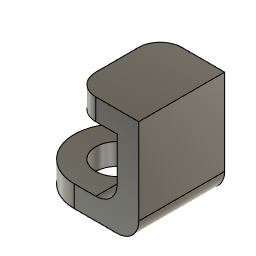
Practice3 (Autodesk Fusion 360 design; units mm, degrees)
Autodesk Fusion 360 part; units mm, degrees
sketch "Sketch1" plane through (0, 0, 0) normal (0, 0, 1) x (1, 0, 0)
  line L0 (0, 0) -> (0, 40)
  line L1 (0, 0) -> (-30, 0)
  line L2 (0, 40) -> (-30, 40)
  circle A0 centre (-30, 20) radius 10
  arc A1 (-30, 40) -> (-30, 0) centre (-30, 20) ccw
  line L3 (0, 0, 0) -> (0, 0, 50.06)
  line L4 (0, 0, 50.06) -> (-30, 0, 50.06)
  line L5 (-30, 0, 50.06) -> (-30, 0, 40.06)
  line L6 (-30, 0, 40.06) -> (-10, 0, 40.06)
  line L7 (-10, 0, 40.06) -> (-10, 0, 10)
  line L8 (-30, 0, 0) -> (-30, 0, 10)
  line L9 (-30, 0, 10) -> (-10, 0, 10)
  line L10 (-10, 0, 10) -> (0, 0, 10)
  dimension "d2" = 30
  dimension "d3" = 40
  dimension "d5" = 30
  dimension "d7" = 20
  dimension "d8" = 20
  dimension "d10" = 50.06
  dimension "d11" = 30
  dimension "d12" = 10
  dimension "d13" = 20
  dimension "d16" = 10
  constraint coincident L0.start L1.start
  constraint vertical L0
  constraint perpendicular L0 L1
  constraint perpendicular L0 L2
  constraint concentric A0 A1
  measures "d2" distance of L0.start L1.end
  measures "d3" distance of L0.start L0.end
  measures "d5" distance of L0.end L2.end
  measures "d7" diameter of A0
  measures "d8" radius of A1
  measures "d10" distance of L0.start L1.start
  measures "d11" distance of L0.start L1.end
  measures "d12" distance of L1.end A1.end
  measures "d16" distance of L1.end A1.end
extrude "Extrude1" add sketch "Sketch1" along normal blind 10 makes body 1
extrude "Extrude2" add sketch "Sketch1" against normal blind 40 contours L3 L4 L5 L6 L7 L10 in plane through (0, 0, 0) normal (0, 1, 0) bodies 1
split "Split1" by plane through (0, 0, 0) normal (0, 1, 0) bodies 1 makes body 2 at (-6.6667, 20, 0)
move_body "Move1" bodies 1 to x (1, 0, 0) y (0, 1, 0) z (0, 0, 1) at (0, 40, 0)
combine "Combine1" operation add target body 1 tool bodies 2
fillet "Fillet1" radius 10 1 edges at (0, 20, 0) on bodies 1
fillet "Fillet2" radius 10 1 edges at (-10, 20, 10) on bodies 1
fillet "Fillet3" radius 10 1 edges at (-30, 40, 45.06) on bodies 1
fillet "Fillet4" radius 10 1 edges at (-30, 0, 45.06) on bodies 1
